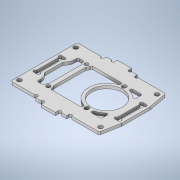
# Autodesk Inventor part: Trunk_chest_horizontal_frame
Saved by Autodesk Inventor 2020.4 (Build 244396000, 396)
## iProperties
Created: 2021-09-09
Part Number: Trunk_chest_horizontal_frame
Material: アルミニウム 2014-T4
Document SubType Name: Modeling
Designer: Masato Kubotera
Density: 2.8 g/cm^3
Appearance: 滑らか - 淡い灰色
Description: A2017 T2
Mass: 6.64657 g
Surface Area: 37.4638 cm^2
Volume: 2.37378 cm^3
Author: Masato Kubotera
Autodesk Inventor part; units mm, degrees
ref_plane "YZ Plane" through (0, 0, 0) normal (1, 0, 0) x (0, 1, 0)
ref_plane "XZ Plane" through (0, 0, 0) normal (0, 1, 0) x (-1, 0, 0)
ref_plane "XY Plane" through (0, 0, 0) normal (0, 0, 1) x (1, 0, 0)
sketch "スケッチ1" plane through (0, 0, 0) normal (0, 0, 1) x (1, 0, 0)
  circle A0 centre (0, 0) radius 11
  line L0 (-25, -19.5) -> (-27, -19.5)
  line L1 (-27, -19.5) -> (-27, -9.5)
  line L2 (-27, -9.5) -> (-25, -9.5)
  circle A1 centre (-13.5, -28) radius 1.35
  arc A2 (-25, -21.6) -> (-25, -19.5) centre (-25, -20.55) ccw
  arc A3 (-25, -9.5) -> (-25, -7.4) centre (-25, -8.45) ccw
  arc A4 (-7.6649, 10.5) -> (-12.9132, 1.5) centre (0, 0) ccw
  arc A5 (-12.52, -3.5) -> (12.52, -3.5) centre (0, 0) ccw
  arc A6 (-11.5, -26.5) -> (-14.5, -25.7087) centre (-13.5, -28) ccw
  line L3 (-14.5, 10.5) -> (-7.6649, 10.5)
  line L4 (-14.5, 10.5) -> (-14.5, 1.5)
  line L5 (-14.5, 1.5) -> (-12.9132, 1.5)
  line L6 (-14.5, -3.5) -> (-12.52, -3.5)
  line L7 (-14.5, -3.5) -> (-14.5, -25.7087)
  line L8 (-35, -44.5) -> (35, -44.5) construction
  line L9 (35, -44.5) -> (35, -39.5) construction
  line L10 (35, -39.5) -> (-35, -39.5) construction
  line L11 (-35, -39.5) -> (-35, -44.5) construction
  line L12 (-35, -44.5) -> (35, -39.5) construction
  line L13 (35, -44.5) -> (-35, -39.5) construction
  line L14 (-35, -42) -> (35, -42) construction
  line L15 (0, -44.5) -> (0, 20.5) construction
  line L16 (-10, 20.5) -> (10, 20.5)
  line L17 (-23.5, -44.5) -> (23.5, -44.5)
  line L18 (-13.5, -1) -> (0, -1) construction
  line L19 (-13.5, -28) -> (-13.5, -1) construction
  circle A7 centre (-20, -42) radius 1.55
  line L20 (-10, -42) -> (10, -42) construction
  line L21 (10, -42) -> (10, -39.5) construction
  line L22 (-10, -39.5) -> (-10, -42) construction
  line L23 (-10, -42) -> (10, -39.5) construction
  line L24 (10, -42) -> (-10, -39.5) construction
  line L25 (-23.5, 18) -> (-10, 20.5)
  line L26 (-10.01, -42.01) -> (10.01, -42.01)
  line L27 (10.01, -42.01) -> (10.01, -39.49)
  line L28 (10.01, -39.49) -> (-10.01, -39.49)
  line L29 (-10.01, -39.49) -> (-10.01, -42.01)
  line L30 (-10.01, -42.01) -> (10.01, -39.49) construction
  line L31 (10.01, -42.01) -> (-10.01, -39.49) construction
  line L32 (-10.01, -40.75) -> (10.01, -40.75) construction
  arc A8 (-10.01, -42.01) -> (-7.91, -42.01) centre (-8.96, -42.01) ccw
  arc A9 (-7.91, -39.49) -> (-10.01, -39.49) centre (-8.96, -39.49) ccw
  line L33 (-35, 13) -> (35, 13) construction
  line L34 (35, 13) -> (35, 18) construction
  line L35 (35, 18) -> (-35, 18) construction
  line L36 (-35, 18) -> (-35, 13) construction
  line L37 (-35, 13) -> (35, 18) construction
  line L38 (35, 13) -> (-35, 18) construction
  line L39 (-35, 15.5) -> (35, 15.5) construction
  circle A10 centre (-20, 15.5) radius 1.55
  line L40 (-10, 15.5) -> (10, 15.5) construction
  line L41 (10, 15.5) -> (10, 18) construction
  line L42 (-10, 18) -> (-10, 15.5) construction
  line L43 (-10, 15.5) -> (10, 18) construction
  line L44 (10, 15.5) -> (-10, 18) construction
  line L45 (-10.01, 15.49) -> (10.01, 15.49)
  line L46 (10.01, 15.49) -> (10.01, 18.01)
  line L47 (10.01, 18.01) -> (-10.01, 18.01)
  line L48 (-10.01, 18.01) -> (-10.01, 15.49)
  line L49 (-10.01, 15.49) -> (10.01, 18.01) construction
  line L50 (10.01, 15.49) -> (-10.01, 18.01) construction
  line L51 (-10.01, 16.75) -> (10.01, 16.75) construction
  arc A11 (-10.01, 15.49) -> (-7.91, 15.49) centre (-8.96, 15.49) ccw
  arc A12 (-7.91, 18.01) -> (-10.01, 18.01) centre (-8.96, 18.01) ccw
  circle A13 centre (13.5, -28) radius 1.35
  arc A14 (12.9132, 1.5) -> (7.6649, 10.5) centre (0, 0) ccw
  line L52 (14.5, 1.5) -> (12.9132, 1.5)
  line L53 (14.5, 10.5) -> (14.5, 1.5)
  line L54 (14.5, 10.5) -> (7.6649, 10.5)
  line L55 (14.5, -3.5) -> (12.52, -3.5)
  circle A15 centre (20, -42) radius 1.55
  line L56 (23.5, 18) -> (10, 20.5)
  arc A16 (7.91, -42.01) -> (10.01, -42.01) centre (8.96, -42.01) ccw
  arc A17 (10.01, -39.49) -> (7.91, -39.49) centre (8.96, -39.49) ccw
  arc A18 (10.01, 18.01) -> (7.91, 18.01) centre (8.96, 18.01) ccw
  arc A19 (7.91, 15.49) -> (10.01, 15.49) centre (8.96, 15.49) ccw
  circle A20 centre (20, 15.5) radius 1.55
  circle A21 centre (-13.5, -1) radius 2.5 construction
  line L57 (-23.5, -28) -> (0, -28) construction
  line L58 (-11.5, -26.5) -> (11.5, -26.5)
  arc A22 (-14.5, -30.2913) -> (-11.5, -29.5) centre (-13.5, -28) ccw
  line L59 (-11.5, -29.5) -> (11.5, -29.5)
  line L60 (-14.5, -30.2913) -> (-14.5, -35.0667)
  line L61 (-14.5, -35.0667) -> (-12.0888, -35.0667)
  line L62 (-6.65, -37.7) -> (6.65, -37.7)
  line L63 (-14.5, -31) -> (0, -31) construction
  arc A23 (-6.65, -37.7) -> (-12.0888, -35.0667) centre (-12.0888, -42) ccw
  line L64 (14.5, -35.0667) -> (12.0888, -35.0667)
  arc A24 (12.0888, -35.0667) -> (6.65, -37.7) centre (12.0888, -42) ccw
  line L65 (-27, -14.5) -> (-13.5, -14.5) construction
  arc A25 (-13, -2.35) -> (-13, 0.35) centre (-13, -1) ccw
  line L66 (-13.5, -2.35) -> (-13, -2.35)
  line L67 (-13, 0.35) -> (-13.5, 0.35)
  arc A26 (-13.5, 0.35) -> (-13.5, -2.35) centre (-13.5, -1) ccw
  arc A27 (13, 0.35) -> (13, -2.35) centre (13, -1) ccw
  line L68 (13.5, -2.35) -> (13, -2.35)
  line L69 (13, 0.35) -> (13.5, 0.35)
  arc A28 (13.5, -2.35) -> (13.5, 0.35) centre (13.5, -1) ccw
  line L70 (-25, -21.6) -> (-25, -25.5)
  line L71 (-25, -25.5) -> (-23.5, -25.5)
  line L72 (-23.5, -27.6) -> (-23.5, -44.5)
  arc A29 (-23.5, -27.6) -> (-23.5, -25.5) centre (-23.5, -26.55) ccw
  line L73 (-25, -7.4) -> (-25, -3.5)
  line L74 (-25, -3.5) -> (-23.5, -3.5)
  arc A30 (-23.5, -3.5) -> (-23.5, -1.4) centre (-23.5, -2.45) ccw
  line L75 (-23.5, -1.4) -> (-23.5, 18)
  line L76 (25, -19.5) -> (27, -19.5)
  line L77 (27, -19.5) -> (27, -9.5)
  line L78 (27, -9.5) -> (25, -9.5)
  arc A31 (25, -19.5) -> (25, -21.6) centre (25, -20.55) ccw
  arc A32 (25, -7.4) -> (25, -9.5) centre (25, -8.45) ccw
  line L79 (25, -21.6) -> (25, -25.5)
  line L80 (23.5, -27.6) -> (23.5, -44.5)
  arc A33 (23.5, -25.5) -> (23.5, -27.6) centre (23.5, -26.55) ccw
  line L81 (25, -3.5) -> (23.5, -3.5)
  arc A34 (23.5, -1.4) -> (23.5, -3.5) centre (23.5, -2.45) ccw
  line L82 (25, -7.4) -> (25, -3.5)
  line L83 (23.5, -1.4) -> (23.5, 18)
  line L84 (25, -25.5) -> (23.5, -25.5)
  line L85 (14.5, -3.5) -> (14.5, -25.7087)
  arc A35 (14.5, -25.7087) -> (11.5, -26.5) centre (13.5, -28) ccw
  arc A36 (11.5, -29.5) -> (14.5, -30.2913) centre (13.5, -28) ccw
  line L86 (14.5, -30.2913) -> (14.5, -35.0667)
  point P0 (0, -42)
  point P1 (0, -40.75)
  point P2 (0, -42)
  point P3 (0, 15.5)
  point P4 (0, 16.75)
  point P5 (0, 15.5)
  point P6 (0, 15.5)
  point P7 (0, 16.75)
  point P8 (7.91, -42.01)
  point P9 (7.91, 15.49)
  point P10 (7.91, 18.01)
  point P11 (-15, -30)
  point P12 (-15, -26)
  dimension "d0" = 22
  dimension "d38" = 2
  dimension "d39" = 10
  dimension "d151" = 1.05
  dimension "d152" = 1.05
  dimension "d171" = 70
  dimension "d172" = 5
  dimension "d173" = 1
  dimension "d176" = 20
  dimension "d177" = 2.5
  dimension "d178" = 2
  dimension "d179" = 2
  dimension "d180" = 1.05
  dimension "d181" = 0.01
  dimension "d182" = 0.01
  dimension "d183" = 3.1
  dimension "d184" = 70
  dimension "d185" = 5
  dimension "d186" = 20
  dimension "d187" = 2.5
  dimension "d188" = 1.05
  dimension "d189" = 0.01
  dimension "d190" = 0.01
  dimension "d191" = 3.1
  dimension "d192" = 52.5
  dimension "d193" = 2.5
  dimension "d194" = 13
  dimension "d195" = 40
  dimension "d196" = 40
  dimension "d199" = 2.7
  dimension "d200" = 2.5
  dimension "d201" = 2.5
  dimension "d204" = 5
  dimension "d206" = 3
  dimension "d207" = 4.0667
  dimension "d208" = 6.7
  dimension "d211" = 13.3
  dimension "d213" = 2.7
  dimension "d214" = 27
  dimension "d215" = 0.5
  dimension "d218" = 1.05
  dimension "d219" = 1.5
  dimension "d220" = 50
  dimension "d221" = 2.5
  dimension "d222" = 27
  dimension "d223" = 3
  dimension "d224" = 22
  constraints: 174 end point, 58 point on circle, 47 horizontal alignment, 37 centre point, 28 midpoint, 23 point on line, 16 equal radius, 15 horizontal, 13 perpendicular, 12 parallel, 11 symmetric about line, 10 tangent, 4 coincident, 4 collinear, 3 concentric, 3 vertical, 15 other
  measures "d0" diameter of A0
  measures "d38" distance of L0.start L0.end
  measures "d39" distance of L0.end L1.end
  measures "d151" radius of A2
  measures "d152" radius of A3
  measures "d171" distance of L10.end L9.end
  measures "d172" distance of L9.end L8.end
  measures "d173" distance of A4.centre L18.end
  measures "d176" distance of L22.start L21.end
  measures "d177" distance of L21.end L20.end
  measures "d178" radial gap between concentric circles of A0 A5
  measures "d179" radial gap between concentric circles of A0 A4
  measures "d180" radius of A8
  measures "d181" horizontal distance of L22.start L28.end
  measures "d182" horizontal distance of L22.start L28.end
  measures "d183" diameter of A7
  measures "d184" distance of L35.end L34.end
  measures "d185" distance of L34.end L33.end
  measures "d186" distance of L44.end L41.end
  measures "d187" distance of L41.end L40.end
  measures "d188" radius of A11
  measures "d189" horizontal distance of L44.end L47.end
  measures "d190" horizontal distance of L44.end L47.end
  measures "d191" diameter of A10
  measures "d192" distance of L33.start L10.end
  measures "d193" distance from line of point (0, 20.5) L35
  measures "d194" distance from line of L33 point (0, 0)
  measures "d195" distance of A15.centre A7.centre
  measures "d196" distance of A20.centre A10.centre
  measures "d199" diameter of A1
  measures "d200" radius of A6
  measures "d201" distance between parallel lines of L33 L3
  measures "d204" diameter of A21
  measures "d206" distance from line of A1.centre L63
  measures "d207" distance of L60.end L63.start
  measures "d208" distance between parallel lines of L63 L62
  measures "d211" distance of L62.start L62.end
  measures "d213" diameter of A25
  measures "d214" distance of L19.start L18.start
  measures "d215" distance of A21.centre A25.centre
  measures "d218" radius of A29
  measures "d219" distance between parallel lines of L72 L70
  measures "d220" distance between parallel lines of L70 L79
  measures "d221" distance from line of L70.end L57
  measures "d222" distance of L19.start A13.centre
  measures "d223" distance between parallel lines of L58 L59
  measures "d224" distance between parallel lines of L74 L71
extrude "押し出し1" add sketch "スケッチ1" along normal blind 2
fillet "フィレット1" radius 1 6 edges at (-23.5, -44.5, 1) (23.5, -44.5, 1) (23.5, 18, 1) (-23.5, 18, 1) (-10, 20.5, 1) (10, 20.5, 1)
fillet "フィレット2" radius 1 24 edges at (-14.5, -35.0667, 1) (-6.65, -37.7, 1) (6.65, -37.7, 1) (-11.5, -26.5, 1) (-11.5, -29.5, 1) (-14.5, -3.5, 1) (-12.52, -3.5, 1) (-12.9132, 1.5, 1) (-14.5, 1.5, 1) (12.52, -3.5, 1) (14.5, 1.5, 1) (12.9132, 1.5, 1) (-7.6649, 10.5, 1) (-14.5, 10.5, 1) (7.6649, 10.5, 1) (14.5, 10.5, 1) (-14.5, -30.2913, 1) (-14.5, -25.7087, 1) (14.5, -25.7087, 1) (14.5, -30.2913, 1) (14.5, -35.0667, 1) (11.5, -29.5, 1) (11.5, -26.5, 1) (14.5, -3.5, 1)
